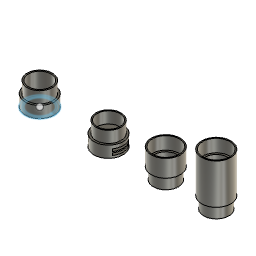
version1 v22 (Autodesk Fusion 360 archive; units mm, degrees)
design "Microscope_cameraAdapter"
Autodesk Fusion 360 part; units mm, degrees
sketch "スケッチ1" plane through (0, 0, 0) normal (0, 0, 1) x (1, 0, 0)
  circle A0 centre (0, 0) radius 10.9
  circle A1 centre (0, 0) radius 9.9
  circle A2 centre (0, 0) radius 11.65
  circle A3 centre (0, 0) radius 12.65
  dimension "d1" = 21.8
  dimension "d2" = -1
  dimension "d8" = 23.3
  dimension "d9" = 1
  constraint coincident A0.centre A1.centre
  constraint concentric A0 A2
  measures "d1" diameter of A0
  measures "d8" diameter of A2
extrude "押し出し3" add sketch "スケッチ1" along normal blind 10 contours A0 makes body 1
sketch "スケッチ2" plane through (0, 0, 10) normal (0, 0, 1) x (-1, 0, 0)
  circle A0 centre (0, 0) radius 9.9
  circle A1 centre (0, 0) radius 10.9
  circle A2 centre (0, 0) radius 11.65
  circle A3 centre (0, 0) radius 12.65
  dimension "d12" = 23.3
  dimension "d13" = 1
  constraint concentric A0 A2
  measures "d12" diameter of A2
extrude "押し出し6" add sketch "スケッチ2" along normal blind 15 separate body contours A3 makes body 2
extrude "押し出し7" add sketch "スケッチ2" along normal blind 4 contours A2 bodies 2 1
extrude "押し出し8" add 1 faces at (10.5261, -0.5415, 10) along direction (0, 0, 1) blind 4 on bodies 2 bodies 2
copy_body "ボディのコピーと貼り付け1" bodies 2 makes body 3
move_body "移動1" bodies 3 to x (1, 0, 0) y (0, 1, 0) z (0, 0, 1) at (44, 0, 0)
extrude "押し出し9" add 1 faces at (31.7304, 0.6285, 25) along direction (0, 0, 1) blind 20 on bodies 3 bodies 3
extrude "押し出し10" add 1 faces at (33.0136, 1.0706, 14) along direction (0, 0, 1) blind 20 on bodies 3 bodies 3
sketch "スケッチ3" plane through (0, 0, 0) normal (0, 0, 1) x (1, 0, 0)
  circle A0 centre (-50, 0) radius 12.65
  circle A1 centre (-50, 0) radius 4
  dimension "d28" = 25.3
  dimension "d29" = 8
  constraint concentric A0 A1
  measures "d28" diameter of A0
  measures "d29" diameter of A1
extrude "押し出し11" add sketch "スケッチ3" along normal blind 10 separate body makes body 4
sketch "スケッチ4" plane through (0, 0, 10) normal (0, 0, 1) x (-1, 0, 0)
  circle A0 centre (50, 0) radius 4
  circle A1 centre (50, 0) radius 12.65
  circle A2 centre (50, 0) radius 10.9
  circle A3 centre (50, 0) radius 9.9
  dimension "d32" = 21.8
  dimension "d33" = -1
  constraint concentric A0 A2
  measures "d32" diameter of A2
extrude "押し出し12" add sketch "スケッチ4" along normal blind 10 contours A2 bodies 4
sketch "スケッチ5" plane through (0, 0, 20) normal (0, 0, 1) x (-1, 0, 0)
  circle A0 centre (50, 0) radius 9.9
  circle A1 centre (50, 0) radius 10.9
  circle A2 centre (50, 0) radius 6.9
  dimension "d36" = 13.8
  constraint concentric A0 A2
  measures "d36" diameter of A2
extrude "押し出し14" add sketch "スケッチ5" along normal blind 1 separate body contours A2 makes body 5
sketch "スケッチ6" plane through (0, 0, 21) normal (0, 0, 1) x (-1, 0, 0)
  circle A0 centre (50, 0) radius 6.9
  line L0 (36.5423, 7) -> (63.4577, 7)
  line L1 (63.4577, 7) -> (63.4577, -7)
  line L2 (63.4577, -7) -> (36.5423, -7)
  line L3 (36.5423, -7) -> (36.5423, 7)
  line L4 (36.5423, 7) -> (63.4577, -7) construction
  line L5 (63.4577, 7) -> (36.5423, -7) construction
  point P0 (50, 0)
  dimension "d41" = 14
  constraint horizontal L0
  constraint perpendicular L0 L1
  constraint parallel L0 L2
  constraint parallel L1 L3
  constraint coincident L4 P0
  constraint coincident L5 P0
  constraint coincident P0 A0.centre
  measures "d41" distance of L0.end L1.end
extrude "押し出し16" add sketch "スケッチ6" along normal blind 2 separate body makes body 6
copy_body "ボディのコピーと貼り付け3" bodies 5 makes body 7
move_body "移動5" bodies 7 to x (1, 0, 0) y (0, 1, 0) z (0, 0, 1) at (0, 0, -19)
combine "結合3" operation cut target body 4 tool bodies 7
extrude "押し出し17" add 1 faces at (-48.074, 1.6384, 21) along direction (0, 0, 1) blind 2 on bodies 5 bodies 5 6
copy_body "ボディのコピーと貼り付け4" bodies 5 makes body 8
move_body "移動6" bodies 8 to x (1, 0, 0) y (0, 1, 0) z (0, 0, 1) at (0, 0, -19)
move_body "移動7" bodies 5 to x (1, 0, 0) y (0, 1, 0) z (0, 0, 1) at (0, 0, -16)
combine "結合4" operation cut target body 4 tool bodies 5 8
sketch "スケッチ7" plane through (0, 0, 0) normal (0, 0, 1) x (1, 0, 0)
  circle A0 centre (-110, 0) radius 9.8
  circle A1 centre (-110, 0) radius 12.65
  circle A2 centre (-110, 0) radius 11
  dimension "d48" = 19.6
  dimension "d49" = 25.3
  dimension "d50" = 22
  constraint concentric A0 A1
  constraint concentric A0 A2
  measures "d48" diameter of A0
  measures "d49" diameter of A1
  measures "d50" diameter of A2
extrude "押し出し19" add sketch "スケッチ7" along normal blind 10 separate body contours A1 makes body 9
extrude "押し出し20" add sketch "スケッチ7" along normal blind 20 contours A2 bodies 9
